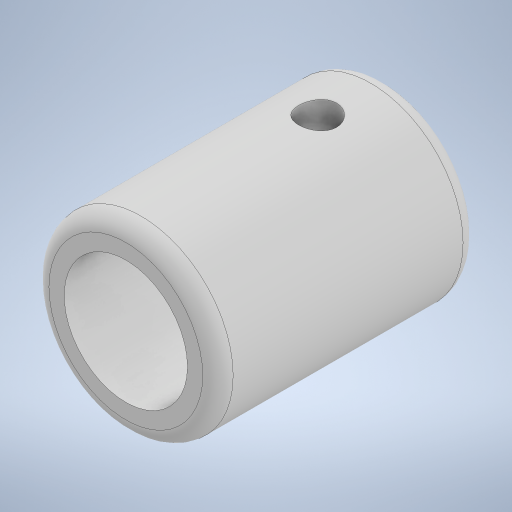
# Autodesk Inventor part: parent_ver.
Saved by Autodesk Inventor 2023 (Build 270158000, 158)
## iProperties
Created: 2023-11-07
Part Number: parent_ver.
Material: 一般
Document SubType Name: Modeling
Designer: bonju
Density: 1 g/cm^3
Appearance: 既定
Author: bonju
Autodesk Inventor part; units mm, degrees
ref_plane "YZ Plane" through (0, 0, 0) normal (1, 0, 0) x (0, 1, 0)
ref_plane "XZ Plane" through (0, 0, 0) normal (0, 1, 0) x (-1, 0, 0)
ref_plane "XY Plane" through (0, 0, 0) normal (0, 0, 1) x (1, 0, 0)
sketch "スケッチ1" plane through (0, 0, 0) normal (0, 0, 1) x (1, 0, 0)
  circle A0 centre (0, 0) radius 4.05
  circle A1 centre (0, 0) radius 6.05
  dimension "d0" = 8.1
  dimension "d1" = 2
  constraints: 2 centre point, 1 coincident
  measures "d0" diameter of A0
  measures "d1" radial gap between concentric circles of A0 A1
extrude "押し出し1" add sketch "スケッチ1" against normal blind 8.1
sketch "スケッチ2" plane through (0, 0, -8.1) normal (0, 0, -1) x (-1, 0, 0)
  circle A0 centre (0, 0) radius 6.05
  circle A1 centre (0, 0) radius 6.05 projected
  dimension "d13" = 0
  constraints: 1 centre point, 1 coincident
  measures "d13" radial gap between concentric circles of A1 A0
extrude "押し出し2" add sketch "スケッチ2" along normal blind 9
sketch "スケッチ3" plane through (0, 0, 0) normal (0, 1, 0) x (-1, 0, 0)
  circle A0 centre (0, -12.6) radius 1.25
  line L0 (4.05, -8.1) -> (-4.05, -8.1) projected
  point P0 (0, 0)
  dimension "d6" = 2.5
  dimension "d7" = 4.5
  constraints: 1 centre point
  measures "d6" diameter of A0
  measures "d7" distance from line of L0 A0.centre
extrude "押し出し3" cut sketch "スケッチ3" along normal through all both and the other way through all
fillet "フィレット1" radius 1 2 edges at (6.05, 0, -17.1) (-6.05, 0, 0)
